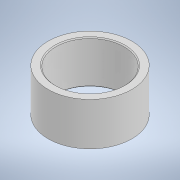
# Autodesk Inventor part: 74. Кольцо распорное
Saved by Autodesk Inventor 2021 (Build 250183000, 183)
## iProperties
Created: 2021-03-11
Part Number: 74. Кольцо распорное
Material: Типовые
Document SubType Name: Modeling
Designer: Данил
Density: 1 g/cm^3
Appearance: По умолчанию
Author: Данил
Autodesk Inventor part; units mm, degrees
ref_plane "YZ Plane" through (0, 0, 0) normal (1, 0, 0) x (0, 1, 0)
ref_plane "XZ Plane" through (0, 0, 0) normal (0, 1, 0) x (-1, 0, 0)
ref_plane "XY Plane" through (0, 0, 0) normal (0, 0, 1) x (1, 0, 0)
sketch "Эскиз1" plane through (0, 0, 0) normal (0, 0, 1) x (1, 0, 0)
  line L0 (0, 11) -> (0, -11)
  line L1 (18, 11) -> (21.5, 11)
  line L2 (21.5, 11) -> (21.5, -11)
  line L3 (21.5, -11) -> (18, -11)
  line L4 (17.5, -10.5) -> (17.5, 10.5)
  line L5 (17.5, 10.5) -> (18, 11)
  line L6 (17.5, -10.5) -> (18, -11)
  point P0 (0, 0)
  point P1 (0, 0)
  point P2 (17.5, 11)
  point P3 (17.5, -11)
  dimension "d0" = 22
  dimension "d1" = 43
  dimension "d2" = 35
  dimension "d3" = 0.5
  dimension "d4" = 45
  dimension "d5" = 0.5
  dimension "d6" = 45
  constraints: 14 end point, 4 point on line, 2 horizontal alignment, 2 parallel, 1 coincident, 1 horizontal, 1 midpoint, 1 perpendicular, 1 vertical
  measures "d0" distance of L0.start L0.end
  measures "d1" diameter of L2 L0
  measures "d2" diameter of L4 L0
  measures "d3" distance of L4.end point (17.5, 11)
  measures "d4" angle of L4 L5
  measures "d5" distance of L4.start point (17.5, -11)
  measures "d6" angle of L4 L6
revolve "Вращение1" add sketch "Эскиз1" angle 360 about axis through (0, 11, 0) along (0, -1, 0)
equation "\"d5\" = d3"
equation "\"d6\" = d4"
